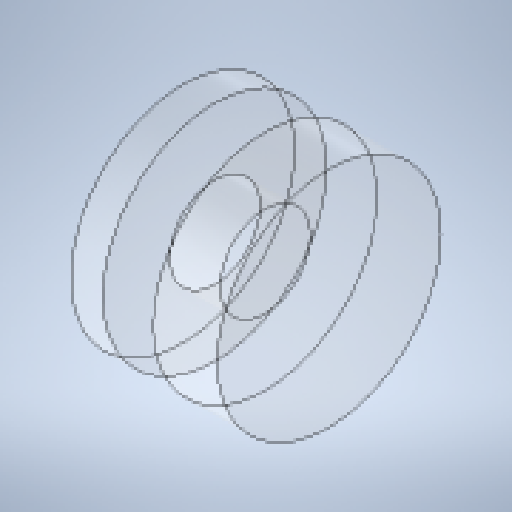
# Autodesk Inventor part: Temp Sprocket
Saved by Autodesk Inventor 2023.4 (Build 274418000, 418)
## iProperties
Created: 2024-05-07
Part Number: Temp Sprocket
Material: Nylon 6/6
Document SubType Name: Modeling
Designer: Nathan Cai
Density: 1.13 g/cm^3
Appearance: Clear - Light
Mass: 25.1453 g
Surface Area: 80.3719 cm^2
Volume: 22.2524 cm^3
Author: Nathan Cai
Autodesk Inventor part; units mm, degrees
ref_plane "YZ Plane" through (0, 0, 0) normal (1, 0, 0) x (0, 1, 0)
ref_plane "XZ Plane" through (0, 0, 0) normal (0, 1, 0) x (-1, 0, 0)
ref_plane "XY Plane" through (0, 0, 0) normal (0, 0, 1) x (1, 0, 0)
sketch "Sketch1" plane through (0, 0, 0) normal (0, 1, 0) x (-1, 0, 0)
  line L0 (0, 0) -> (10, 0)
  line L1 (10, 0) -> (10, -9)
  line L2 (10, -9) -> (0, -9)
  line L3 (0, -9) -> (0, 0)
  line L4 (10, 0) -> (16.35, 0)
  line L5 (16.35, 0) -> (16.35, -22.225)
  line L6 (16.35, -22.225) -> (10, -22.225)
  line L7 (10, -22.225) -> (10, 0)
  line L8 (0, 0) -> (-12.7, 0)
  line L9 (-12.7, 0) -> (-12.7, -22.225)
  line L10 (-12.7, -22.225) -> (0, -22.225)
  line L11 (0, -22.225) -> (0, 0)
  point P0 (0, -9)
  point P1 (10, -9)
  dimension "d0" = 10
  dimension "d1" = 9
  dimension "d2" = 6.35
  dimension "d3" = 22.225
  dimension "d4" = 22.225
  dimension "d5" = 12.7
  constraints: 24 end point, 6 parallel, 3 horizontal, 3 perpendicular
  measures "d0" distance of L1.end L2.end
  measures "d1" distance of L0.end L1.end
  measures "d2" distance of L5.end L6.end
  measures "d3" distance of L4.end L5.end
  measures "d4" distance of L8.end L9.end
  measures "d5" distance of L9.end L10.end
revolve "Revolution1" add sketch "Sketch1" angle 360 about axis through (0, 0, 0) along (-1, 0, 0)
equation "\"d4\" = d3"
body "Solid1"
